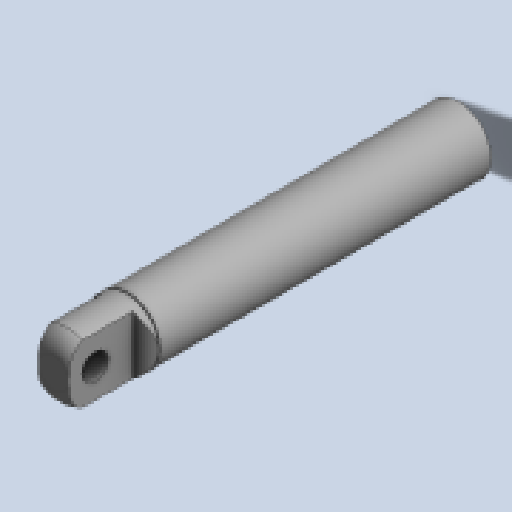
# Autodesk Inventor part: 1610-50H-2KG-12V-B07-Shaft
Saved by Autodesk Inventor 2025.2 (Build 292293000, 293)
## iProperties
Created: 2026-01-24
Part Number: 1610-50H-2KG-12V-B07-Shaft
Material: Generic
Document SubType Name: Modeling
Designer: valer
Density: 1 g/cm^3
Appearance: Default
Author: valer
Autodesk Inventor part; units mm, degrees
ref_plane "YZ Plane" through (0, 0, 0) normal (1, 0, 0) x (0, 1, 0)
ref_plane "XZ Plane" through (0, 0, 0) normal (0, 1, 0) x (-1, 0, 0)
sketch "Rod" plane through (0, 0, 0) normal (0, 0, 1) x (1, 0, 0)
  circle A0 centre (0, 0) radius 5
  dimension "d0" = 10
  constraints: 1 centre point, 1 coincident
  measures "d0" diameter of A0
extrude "RodFeature" add sketch "Rod" along normal blind 50.5
ref_plane "RodEndPlane" through (0, 0, 50.5) normal (0, 0, 1) x (1, 0, 0)
sketch "RodEnd" plane through (0, 0, 50.5) normal (0, 0, 1) x (1, 0, 0)
  circle A0 centre (0, 0) radius 5 projected
extrude "RodEndFeature" add sketch "RodEnd" along normal blind 11
sketch "RodEndTip" plane through (0, 0, 0) normal (1, 0, 0) x (0, 1, 0)
  line L0 (5, 0) -> (5, 61.5)
  line L1 (5, 61.5) -> (-5, 61.5)
  line L2 (-5, 0) -> (-5, 61.5)
  arc A0 (5, 59.5) -> (2, 61.5) centre (2.169876, 58.504813) ccw
  line L3 (0, -12.300193) -> (0, 73.801157) construction
  arc A1 (-2, 61.5) -> (-5, 59.5) centre (-2.169876, 58.504813) ccw
  point P0 (0, 0)
  point P1 (-5, 59.5)
  point P2 (-2.339751, 61.5)
  point P3 (2.339751, 61.5)
  dimension "d6" = 3
  dimension "d7" = 2
  dimension "d8" = 3
  constraints: 4 point on circle, 3 symmetric about line, 2 centre point, 2 point on line, 1 other
  measures "d6" horizontal distance of A0.end A0.start
  measures "d7" distance of L0.end A0.start
  measures "d8" radius of A0
sketch "RodEndTip outline for RodEndTipFeature" plane through (0, 0, 0) normal (1, 0, 0) x (0, 1, 0)
  arc A0 (-5, 59.5) -> (-2.339751, 61.5) centre (-2.169876, 58.504813) cw
  line L0 (-5, 61.5) -> (-5, 59.5)
  line L1 (-2.339751, 61.5) -> (-5, 61.5)
  arc A1 (2.339751, 61.5) -> (5, 59.5) centre (2.169876, 58.504813) cw
  line L2 (5, 61.5) -> (2.339751, 61.5)
  line L3 (5, 59.5) -> (5, 61.5)
revolve "RodEndTipFeature" cut sketch "RodEndTip outline for RodEndTipFeature" angle 360 about axis through (0, 0, -10) along (0, 0, 1)
sketch "RodEndProfile" plane through (0, 0, 0) normal (0, 1, 0) x (-1, 0, 0)
  line L0 (2.339751, 61.5) -> (-2.339751, 61.5)
  line L1 (-5, 59.5) -> (5, 59.5)
  line L2 (-5, 59.5) -> (5, 59.5)
  line L3 (5, 0) -> (-5, 0)
  line L4 (-2.339751, 61.5) -> (2.339751, 61.5)
  line L5 (2.339751, 61.5) -> (2.339751, 50.5)
  line L6 (2.339751, 50.5) -> (-2.339751, 50.5)
  line L7 (-2.339751, 50.5) -> (-2.339751, 61.5)
  line L8 (-7.423886, 50.5) -> (7.423886, 50.5)
  arc A0 (-2.339751, 61.5) -> (-5, 59.5) centre (-2.169876, 58.504813) ccw
  arc A1 (5, 59.5) -> (2.339751, 61.5) centre (2.169876, 58.504813) ccw
  line L9 (5, 0) -> (5, 59.5)
  line L10 (-5, 0) -> (-5, 59.5)
  arc A2 (5, 50.5) -> (2.339751, 51.83) centre (2.339751, 48.504503) ccw
  line L11 (0, -12.280546) -> (0, 73.683275)
  arc A3 (-2.339751, 51.83) -> (-5, 50.5) centre (-2.339751, 48.504503) ccw
  line L12 (2.339751, 51.83) -> (-2.339751, 51.83) construction
  point P0 (0, 0)
  point P1 (5, 50)
  point P2 (-2.339751, 51.83)
  dimension "d10" = 4.6795
  dimension "d13" = 1.33
  constraints: 10 end point, 4 point on circle, 4 point on line, 3 symmetric about line, 2 centre point, 2 horizontal, 2 parallel, 1 collinear, 1 perpendicular, 1 tangent, 1 other
  measures "d10" distance between parallel lines of L5 L7
  measures "d13" distance between parallel lines of L6 L12
extrude "RodEndProfileFeature" cut sketch "RodEndProfile" along normal through all both and the other way through all contours A1 L1 L5 | L1 L9 A2 L5 | L7 L1 A0 | L7 A3 L10 L1
sketch "RodEndEtch" plane through (0, 0, 50.5) normal (0, 0, 1) x (1, 0, 0)
  circle A0 centre (0, 0) radius 5 projected
  circle A1 centre (0, 0) radius 4.75
  dimension "d14" = 0.25
  constraints: 1 centre point, 1 coincident
  measures "d14" radial gap between concentric circles of A1 A0
extrude "RodEndEtchFeature" cut sketch "RodEndEtch" against normal blind 0.25
sketch "RodEndHole" plane through (2.339751, -4.418774, 51.83) normal (1, 0, 0) x (0, 0, -1)
  line L0 (64.130968, 4.418774) -> (-21.975807, 4.418774) construction
  line L1 (-3.67, 6.418774) -> (-7.67, 6.418774)
  line L2 (-7.67, 6.418774) -> (-7.67, 2.418774)
  line L3 (-7.67, 2.418774) -> (-3.67, 2.418774)
  line L4 (-3.67, 2.418774) -> (-3.67, 6.418774)
  line L5 (-3.67, 6.418774) -> (-7.67, 2.418774) construction
  line L6 (-7.67, 6.418774) -> (-3.67, 2.418774) construction
  line L7 (-9.67, 4.418774) -> (-9.67, 2.079023)
  point P0 (51.83, 4.418774)
  point P1 (-5.67, 4.418774)
  dimension "d17" = 2
  dimension "d18" = 4
  constraints: 12 end point, 2 midpoint, 2 parallel, 2 perpendicular, 1 horizontal, 1 point on line
  measures "d17" distance between parallel lines of L7 L2
  measures "d18" distance of L1.end L2.end
hole "RodEndHoleFeature" at (2.339751, 0, 57.5) direction (-1, 0, 0) diameter 4 end through all
body "Solid1"
